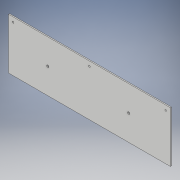
# Autodesk Inventor part: Drive Side Inner Plate
Saved by Autodesk Inventor 2017 (Build 210142000, 142)
## iProperties
Created: 2017-10-12
Part Number: Drive Side Inner Plate
Material: Generic
Document SubType Name: Modeling
Designer: Kenneth
Density: 1 g/cm^3
Appearance: Default
Author: Kenneth
Autodesk Inventor part; units mm, degrees
ref_plane "YZ Plane" through (0, 0, 0) normal (1, 0, 0) x (0, 1, 0)
ref_plane "XZ Plane" through (0, 0, 0) normal (0, 1, 0) x (-1, 0, 0)
ref_plane "XY Plane" through (0, 0, 0) normal (0, 0, 1) x (1, 0, 0)
sketch "Sketch1" plane through (0, 0, 0) normal (0, 0, 1) x (1, 0, 0)
  line L0 (-222.25, -69.85) -> (222.25, -69.85)
  line L1 (222.25, -69.85) -> (222.25, 69.85)
  line L2 (222.25, 69.85) -> (-222.25, 69.85)
  line L3 (-222.25, 69.85) -> (-222.25, -69.85)
  line L4 (-222.25, -69.85) -> (222.25, 69.85) construction
  line L5 (222.25, -69.85) -> (-222.25, 69.85) construction
  point P0 (0, 0)
  dimension "d0" = 444.5
  dimension "d1" = 139.7
  constraints: 12 end point, 2 midpoint, 2 parallel, 1 horizontal, 1 perpendicular
  measures "d0" distance of L1.end L2.end
  measures "d1" distance of L0.end L1.end
extrude "Extrusion1" add sketch "Sketch1" along normal blind 3.175
sketch "Sketch2" plane through (0, 0, 3.175) normal (0, 0, 1) x (1, 0, 0)
  circle A0 centre (209.55, 57.15) radius 2.286
  line L0 (222.25, -69.85) -> (222.25, 69.85) projected
  line L1 (222.25, 69.85) -> (-222.25, 69.85) projected
  circle A1 centre (-209.55, 57.15) radius 2.286
  line L2 (-222.25, 69.85) -> (-222.25, -69.85) projected
  circle A2 centre (0, 57.15) radius 2.286
  point P0 (0, 0)
  dimension "d10" = 4.572
  dimension "d12" = 12.7
  dimension "d11" = 12.7
  dimension "d7" = 4.572
  dimension "d9" = 12.7
  dimension "d8" = 12.7
  dimension "d5" = 4.572
  dimension "d6" = 12.7
  constraints: 3 centre point
  measures "d10" diameter of A0
  measures "d12" distance from line of L0 A0.centre
  measures "d11" distance from line of L1 A0.centre
  measures "d7" diameter of A1
  measures "d9" distance from line of L2 A1.centre
  measures "d8" distance from line of L1 A1.centre
  measures "d5" diameter of A2
  measures "d6" distance from line of L1 A2.centre
extrude "Extrusion2" cut sketch "Sketch2" against normal blind 3.175
sketch "Sketch3" plane through (0, 0, 3.175) normal (0, 0, 1) x (1, 0, 0)
  circle A0 centre (-114.3, 0) radius 2.9972
  circle A1 centre (107.95, 0) radius 2.9972
  line L0 (-222.25, 69.85) -> (-222.25, -69.85) projected
  line L1 (222.25, -69.85) -> (222.25, 69.85) projected
  line L2 (-222.25, -69.85) -> (222.25, -69.85) projected
  point P0 (0, 0)
  dimension "d16" = 5.9944
  dimension "d17" = 5.9944
  dimension "d18" = 107.95
  dimension "d19" = 114.3
  dimension "d20" = 69.85
  constraints: 2 centre point
  measures "d16" diameter of A0
  measures "d17" diameter of A1
  measures "d18" distance from line of L0 A0.centre
  measures "d19" distance from line of L1 A1.centre
  measures "d20" distance from line of L2 A1.centre
extrude "Extrusion3" cut sketch "Sketch3" against normal blind 25.4
body "Solid1"
